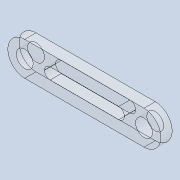
# Autodesk Inventor part: ウィングおさえ
Saved by Autodesk Inventor 2020 (Build 240168000, 168)
## iProperties
Part Number: ウィングおさえ
Material: ポリカーボネート、クリア
Document SubType Name: Modeling
Designer: 原知也
Density: 1.2 g/cm^3
Appearance: ポリカーボネート - クリア
Mass: 0.288853 g
Surface Area: 4.76836 cm^2
Volume: 0.240711 cm^3
Author: 原知也
Autodesk Inventor part; units mm, degrees
ref_plane "YZ Plane" through (0, 0, 0) normal (1, 0, 0) x (0, 1, 0)
ref_plane "XZ Plane" through (0, 0, 0) normal (0, 1, 0) x (-1, 0, 0)
ref_plane "XY Plane" through (0, 0, 0) normal (0, 0, 1) x (1, 0, 0)
sketch "スケッチ1" plane through (0, 0, 0) normal (0, 1, 0) x (-1, 0, 0)
  circle A0 centre (0, 0) radius 1.5
  line L0 (0, 0) -> (-21.2, 0) construction
  circle A1 centre (-21.2, 0) radius 1.5
  line L1 (0, 0) -> (-21.2, 0) construction
  line L2 (0, 3) -> (-21.2, 3)
  line L3 (-21.2, -3) -> (0, -3)
  arc A2 (0, -3) -> (0, 3) centre (0, 0) ccw
  arc A3 (-21.2, 3) -> (-21.2, -3) centre (-21.2, 0) ccw
  point P0 (-10.6, 0)
  dimension "d0" = 3
  dimension "d1" = 3
  dimension "d2" = 21.2
  dimension "d3" = 6
  constraints: 10 end point, 4 centre point, 4 point on circle, 4 tangent, 2 coincident, 2 horizontal, 1 midpoint, 1 parallel
  measures "d0" diameter of A0
  measures "d1" diameter of A1
  measures "d2" distance of L0.start L0.end
  measures "d3" diameter of A3
extrude "押し出し1" add sketch "スケッチ1" along normal blind 2
sketch "スケッチ2" plane through (0, 2, 0) normal (0, 1, 0) x (1, 0, 0)
  circle A0 centre (21.2, 0) radius 1.5 projected
  circle A1 centre (0, 0) radius 1.5 projected
  line L0 (0, -3) -> (21.2, -3) projected
  arc A2 (21.2, -3) -> (21.2, 3) centre (21.2, 0) ccw projected
  line L1 (21.2, 3) -> (0, 3) projected
  arc A3 (0, 3) -> (0, -3) centre (0, 0) ccw projected
  line L2 (3.3481, 1.02) -> (17.8519, 1.02)
  arc A4 (21.2, -1.5) -> (21.2, 1.5) centre (21.2, 0) ccw
  line L3 (17.8519, -1.02) -> (3.3481, -1.02)
  arc A5 (0, 1.5) -> (0, -1.5) centre (0, 0) ccw
  arc A6 (17.8519, 1.02) -> (17.8519, -1.02) centre (21.2, 0) ccw
  arc A7 (3.3481, -1.02) -> (3.3481, 1.02) centre (0, 0) ccw
  line L4 (0, -3) -> (21.2, -3) projected
  dimension "d8" = 1.98
  dimension "d12" = 1.98
  dimension "d13" = 2
  dimension "d14" = 2
  constraints: 8 point on circle, 4 centre point, 4 end point, 2 coincident, 1 parallel
  measures "d8" distance between parallel lines of L1 L2
  measures "d12" distance between parallel lines of L0 L3
  measures "d13" radial gap between concentric circles of A7 A1
  measures "d14" radial gap between concentric circles of A6 A0
extrude "押し出し2" cut sketch "スケッチ2" against normal blind 2 contours L2 A6 L3 A7
fillet "フィレット1" radius 1 4 edges at (3.3481, 1, 1.02) (3.3481, 1, -1.02) (17.8519, 1, 1.02) (17.8519, 1, -1.02)
